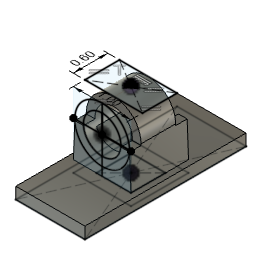
Preparation_1.1 v1 (Autodesk Fusion 360 design; units mm, degrees)
Autodesk Fusion 360 part; units mm, degrees
note: some values were not read from the file. Set by a fixed rule: which sketch regions a step uses.
sketch "Sketch1" plane through (0, 0, 0) normal (0, 0, 1) x (1, 0, 0)
sketch "Sketch2" plane through (0, 0, 0) normal (0, 0, 1) x (1, 0, 0)
  line L0 (6, 14) -> (-6, 14)
  line L1 (-6, 14) -> (-6, -14)
  line L2 (-6, -14) -> (6, -14)
  line L3 (6, -14) -> (6, 14)
  line L4 (6, 14) -> (-6, -14) construction
  line L5 (-6, 14) -> (6, -14) construction
  line L6 (-3, 3) -> (3, 3)
  line L7 (3, 3) -> (3, -3)
  line L8 (3, -3) -> (-3, -3)
  line L9 (-3, -3) -> (-3, 3)
  line L10 (-3, 3) -> (3, -3) construction
  line L11 (3, 3) -> (-3, -3) construction
  line L12 (5, -5) -> (-5, -5)
  line L13 (-5, -5) -> (-5, 5)
  line L14 (-5, 5) -> (5, 5)
  line L15 (5, 5) -> (5, -5)
  dimension "d10" = 12
  dimension "d11" = 28
  dimension "d12" = 6
  dimension "d13" = 6
  dimension "d14" = -2
  constraint horizontal L0
  constraint perpendicular L0 L1
  constraint parallel L0 L2
  constraint parallel L1 L3
  constraint coincident L4 origin
  constraint coincident L5 origin
  constraint horizontal L6
  constraint perpendicular L6 L7
  constraint parallel L6 L8
  constraint parallel L7 L9
  constraint coincident L10 origin
  constraint coincident L11 origin
  measures "d10" distance of L1.end L2.end
  measures "d11" distance of L0.end L1.end
  measures "d12" distance of L7.end L8.end
  measures "d13" distance of L6.end L7.end
extrude "Extrude3" add sketch "Sketch2" along normal blind 2 contours L0 L1 L2 L3 | L6 L7 L8 L9 | L12 L13 L14 L15
extrude "Extrude4" add sketch "Sketch2" along normal blind 13 contours L6 L7 L8 L9 | L12 L13 L14 L15
extrude "Extrude5" cut sketch "Sketch2" along normal blind 9.5 contours L6 L7 L8 L9
sketch "Sketch3" plane through (0, -5, 0) normal (0, -1, 0) x (1, 0, 0)
  line L0 (-5, 2) -> (5, 2)
  line L1 (5, 2) -> (5, 13)
  line L2 (5, 13) -> (-5, 13)
  line L3 (-5, 13) -> (-5, 2)
  line L4 (0, 13) -> (0, 11.5)
  line L5 (0, 11.5) -> (0, 5)
  line L6 (0, 5) -> (0, 2)
  line L7 (0, 11.5) -> (0, 8.25)
  circle A0 centre (0, 8.25) radius 3.25
  circle A1 centre (0, 8.25) radius 4.75
  line L8 (0, 8.25) -> (5, 8.25)
  line L9 (5, 8.25) -> (-5, 8.25)
  dimension "d21" = 1.5
  dimension "d22" = 6.5
  dimension "d23" = 3.25
  dimension "d24" = 6.5
  dimension "d25" = 1.5
  constraint midpoint L2 L4.start
  constraint perpendicular L2 L4
  constraint perpendicular L2 L5
  constraint midpoint L0 L6.end
  constraint perpendicular L2 L7
  constraint coincident L7.end A0.centre
  constraint coincident L1 L8.end
  constraint perpendicular L1 L8
  constraint coincident L3 L9.end
  constraint perpendicular L3 L9
  measures "d21" distance of L4.start L4.end
  measures "d22" distance of L4.end L5.end
  measures "d23" distance of L4.end L7.end
  measures "d24" diameter of A0
extrude "Extrude6" cut sketch "Sketch3" against normal blind 12 contours L5 A0 L9 | L5 A0 L8 L9 | L5 L7 A0 L9 | L5 L7 A0 L8 L9
extrude "Extrude7" cut sketch "Sketch3" against normal blind 10 contours L2 L3 A1 L9 | L1 L2 A1 L8 L9
sketch "Sketch4" plane through (0, 5, 0) normal (0, 1, 0) x (-1, 0, 0)
  line L0 (-4.75, 8.25) -> (-5, 8.25)
  line L1 (-5, 8.25) -> (-5, 2)
  line L2 (-5, 2) -> (5, 2)
  line L3 (5, 2) -> (5, 8.25)
  line L4 (5, 8.25) -> (4.75, 8.25)
  arc A0 (4.75, 8.25) -> (-4.75, 8.25) centre (0, 8.25) ccw
  circle A1 centre (0, 8.25) radius 3.25
  line L5 (4.75, 8.25) -> (5, 2)
  line L6 (-5, 2) -> (-4.75, 8.25)
  constraint coincident L4.end A0.start
  constraint coincident L2.end L3.start
  constraint coincident L1.end L2.start
  constraint coincident L0.start A0.end
extrude "Extrude8" cut sketch "Sketch4" against normal blind 10 contours L0 L1 L6 | L3 L4 L5
sketch "Sketch5" plane through (0, 0, 0) normal (0, 0, 1) x (1, 0, 0)
  line L0 (3, 3) -> (-3, 3)
  line L1 (-3, 3) -> (-3, -3)
  line L2 (-3, -3) -> (3, -3)
  line L3 (3, -3) -> (3, 3)
  line L4 (3, 3) -> (-3, -3) construction
  line L5 (-3, 3) -> (3, -3) construction
  dimension "d32" = 6
  dimension "d33" = 6
  constraint horizontal L0
  constraint perpendicular L0 L1
  constraint parallel L0 L2
  constraint parallel L1 L3
  constraint coincident L4 origin
  constraint coincident L5 origin
  measures "d32" distance of L1.end L2.end
  measures "d33" distance of L0.end L1.end
ref_plane "WorkPlane1" through (0, 0, 13) normal (0, 0, 1) x (1, 0, 0)
sketch "Sketch6" plane through (0, 0, 13) normal (0, 0, 1) x (1, 0, 0)
  line L0 (5, 3) -> (-5, 3)
  line L1 (-5, 3) -> (-5, -3)
  line L2 (-5, -3) -> (5, -3)
  line L3 (5, -3) -> (5, 3)
  line L4 (5, 3) -> (-5, -3) construction
  line L5 (-5, 3) -> (5, -3) construction
  dimension "d35" = 10
  dimension "d36" = 6
  constraint horizontal L0
  constraint perpendicular L0 L1
  constraint parallel L0 L2
  constraint parallel L1 L3
  constraint coincident L4 origin
  constraint coincident L5 origin
  measures "d35" distance of L1.end L2.end
  measures "d36" distance of L0.end L1.end
sketch "Sketch7" plane through (0, 0, 13) normal (0, 0, 1) x (1, 0, 0)
  line L0 (-5, 5) -> (5, 5)
  line L1 (5, 5) -> (5, -5)
  line L2 (5, -5) -> (-5, -5)
  line L3 (-5, -5) -> (-5, 5)
  line L4 (-5, 5) -> (5, -5) construction
  line L5 (5, 5) -> (-5, -5) construction
  line L6 (5, -5) -> (-5, -5)
  line L7 (-5, -5) -> (-5, -3)
  line L8 (-5, -3) -> (5, -3)
  line L9 (5, -3) -> (5, -5)
  line L10 (5, 5) -> (5, 5)
  line L11 (5, 5) -> (5, 3)
  line L12 (5, 3) -> (5, 3)
  line L13 (5, 3) -> (5, 5)
  line L14 (-5, 3.0009) -> (5, 3.0009)
  line L15 (5, 3.0009) -> (5, 5)
  line L16 (5, 5) -> (-5, 5)
  line L17 (-5, 5) -> (-5, 3.0009)
  dimension "d37" = 10
  constraint horizontal L0
  constraint perpendicular L0 L1
  constraint parallel L0 L2
  constraint parallel L1 L3
  constraint coincident L4 origin
  constraint coincident L5 origin
  constraint horizontal L6
  constraint vertical L7
  constraint horizontal L8
  constraint vertical L9
  constraint coincident L3 L7.end
  constraint vertical L11
  constraint vertical L13
  constraint coincident L1 L11.end
  constraint horizontal L14
  constraint vertical L15
  constraint horizontal L16
  constraint vertical L17
  constraint coincident L3 L14.start
  measures "d37" distance of L1.end L2.end
extrude "Extrude9" cut sketch "Sketch7" against normal blind 5 contours L0 L1 L3 L11 L13 L14 L15 L16 L17 | L1 L2 L3 L6 L7 L8 L9
